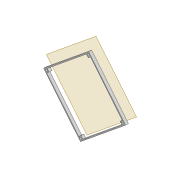
# Autodesk Inventor part: Stage_shunt
Saved by Autodesk Inventor 2020 (Build 240168000, 168)
## iProperties
Created: 2022-05-23
Part Number: Stage_shunt
Material: Generic
Document SubType Name: Modeling
Designer: CDT
Density: 1 g/cm^3
Appearance: Default
Author: CDT
Autodesk Inventor part; units mm, degrees
ref_plane "YZ Plane" through (0, 0, 0) normal (1, 0, 0) x (0, 1, 0)
ref_plane "XZ Plane" through (0, 0, 0) normal (0, 1, 0) x (-1, 0, 0)
ref_plane "XY Plane" through (0, 0, 0) normal (0, 0, 1) x (1, 0, 0)
ref_plane "Work Plane1" through (-43.297, -16.1171, -34.8261) normal (0, 0, 1) x (0.7744854, 0.6325917, 0)
sketch "Sketch1" plane through (-43.297, -16.1171, -34.8261) normal (0, 0, 1) x (0.7744854, 0.6325917, 0)
  line L0 (-79.4504, 49.077) -> (40.5496, 49.077)
  line L1 (40.5496, 49.077) -> (40.5496, -70.923)
  line L2 (40.5496, -70.923) -> (-79.4504, -70.923)
  line L3 (-79.4504, -70.923) -> (-79.4504, 49.077)
  line L4 (-77.4504, 47.077) -> (38.5496, 47.077)
  line L5 (38.5496, 47.077) -> (38.5496, -68.923)
  line L6 (38.5496, -68.923) -> (-77.4504, -68.923)
  line L7 (-77.4504, -68.923) -> (-77.4504, 47.077)
  line L8 (-79.4504, 49.077) -> (-71.4504, 49.077)
  line L9 (-71.4504, 49.077) -> (-71.4504, 41.077)
  line L10 (-71.4504, 41.077) -> (-79.4504, 41.077)
  line L11 (-79.4504, 41.077) -> (-79.4504, 49.077)
  line L12 (40.5496, 49.077) -> (32.5496, 49.077)
  line L13 (32.5496, 49.077) -> (32.5496, 41.077)
  line L14 (32.5496, 41.077) -> (40.5496, 41.077)
  line L15 (40.5496, 41.077) -> (40.5496, 49.077)
  line L16 (-79.4504, -70.923) -> (-71.4504, -70.923)
  line L17 (-71.4504, -70.923) -> (-71.4504, -62.923)
  line L18 (-71.4504, -62.923) -> (-79.4504, -62.923)
  line L19 (-79.4504, -62.923) -> (-79.4504, -70.923)
  line L20 (40.5496, -70.923) -> (32.5496, -70.923)
  line L21 (32.5496, -70.923) -> (32.5496, -62.923)
  line L22 (32.5496, -62.923) -> (40.5496, -62.923)
  line L23 (40.5496, -62.923) -> (40.5496, -70.923)
  circle A0 centre (-75.4504, 45.077) radius 2
  circle A1 centre (36.5496, 45.077) radius 2
  circle A2 centre (-75.4504, -66.923) radius 2
  circle A3 centre (36.5496, -66.923) radius 2
  point P0 (43.7284, -14.9068)
  point P1 (-71.4504, 47.077)
  point P2 (32.5496, 47.077)
  point P3 (38.5496, 41.077)
  point P4 (38.5496, -62.923)
  point P5 (32.5496, -68.923)
  point P6 (-71.4504, -68.923)
  point P7 (-77.4504, -62.923)
  point P8 (-77.4504, 41.077)
  dimension "d0" = 2
  dimension "d1" = 120
  dimension "d2" = 120
  dimension "d3" = 8
  dimension "d4" = 8
  dimension "d5" = 8
  dimension "d6" = 8
  dimension "d7" = 8
  dimension "d8" = 8
  dimension "d9" = 8
  dimension "d10" = 8
  dimension "d11" = 4
  dimension "d12" = 4
  dimension "d13" = 4
  dimension "d14" = 4
  dimension "d15" = 4
  dimension "d16" = 4
  dimension "d17" = 4
  dimension "d18" = 4
  dimension "d19" = 4
  dimension "d20" = 4
  dimension "d21" = 4
  dimension "d22" = 4
  constraints: 48 end point, 12 parallel, 6 perpendicular, 5 horizontal, 4 centre point, 3 other
  measures "d0" distance between parallel lines of L3 L7
  measures "d1" distance of L1.end L2.end
  measures "d2" distance of L2.end L0.start
  measures "d3" distance of L9.end L10.end
  measures "d4" distance of L8.end L9.end
  measures "d5" distance of L14.end L13.end
  measures "d6" distance of L13.end L12.end
  measures "d7" distance of L18.end L17.end
  measures "d8" distance of L17.end L16.end
  measures "d9" distance of L21.end L22.end
  measures "d10" distance of L20.end L21.end
  measures "d11" diameter of A0
  measures "d12" diameter of A1
  measures "d13" diameter of A2
  measures "d14" diameter of A3
  measures "d15" distance from line of L2 A3.centre
  measures "d16" distance from line of L1 A3.centre
  measures "d17" distance from line of L0 A1.centre
  measures "d18" distance from line of L1 A1.centre
  measures "d19" distance from line of L0 A0.centre
  measures "d20" distance from line of L11 A0.centre
  measures "d21" distance from line of L3 A2.centre
  measures "d22" distance from line of L2 A2.centre
extrude "Extrusion1" add sketch "Sketch1" along normal blind 6 contours L0 L9 L4 L7 L10 L3 | L0 L13 L4 L9 | L10 L7 L18 L3 | L0 L1 L14 L5 L4 L13 | L9 L10 L7 A0 L4 | L18 L7 L6 L17 L2 L3 | L4 A1 L5 L14 L13 | A0 L7 L4 | L18 L17 L6 A2 L7 | L1 L22 L5 L14 | L4 L5 A1 | L17 L6 L21 L2 | A2 L6 L7 | L1 L2 L21 L6 L5 L22 | L5 A3 L6 L21 L22 | L5 L6 A3
equation "\"d2\" = d1"
equation "\"d3\" = d6"
equation "\"d4\" = d6"
equation "\"d5\" = d6"
equation "\"d7\" = d6"
equation "\"d8\" = d6"
equation "\"d9\" = d6"
equation "\"d10\" = d6"
equation "\"d15\" = d18"
equation "\"d16\" = d17"
equation "\"d18\" = d17"
equation "\"d19\" = d17"
equation "\"d20\" = d17"
equation "\"d21\" = d17"
equation "\"d22\" = d17"
body "Solid1"
